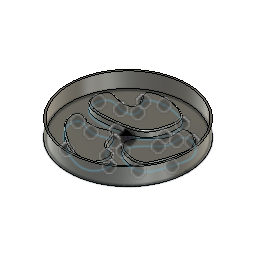
TreeCircleNatural (Autodesk Fusion 360 design; units mm, degrees)
part number: 2026-04-19-12-51-08-975
Autodesk Fusion 360 part; units mm, degrees
sketch "Sketch1" plane through (0, 0, 0) normal (0, 0, 1) x (1, 0, 0)
  circle A0 centre (0, 0) radius 49.5
  circle A1 centre (0, 0) radius 51
  spline S0 degree 5 poles (-8.877426, 39.65922) (-9.821768, 39.602929) (-11.679978, 39.421488) (-14.327292, 38.942346) (-17.354011, 37.914724) (-19.766072, 36.123006) (-20.47548, 33.984554) (-19.509504, 31.627397) (-17.465934, 29.079171) (-15.289166, 26.333804) (-13.947888, 23.4551) (-14.174667, 20.647723) (-16.111086, 18.392073) (-19.407676, 17.242742) (-23.484994, 17.496021) (-27.731291, 18.922825) (-31.751181, 20.409062) (-35.299448, 20.440773) (-38.087025, 18.002518) (-39.766856, 12.861128) (-39.522082, 7.230355) (-37.012223, 2.740009) (-32.437721, -0.082363) (-26.301826, -1.236337) (-19.307435, -1.150796) (-12.19163, -0.372936) (-5.599879, 0.626949) (0.088492, 1.75897) (4.753453, 3.267551) (8.436375, 5.503794) (11.276045, 8.784755) (13.420412, 13.149702) (14.974017, 18.315391) (15.867055, 23.150729) (16.029964, 27.116416) (15.41933, 30.175326) (14.008136, 32.541013) (11.793651, 34.522624) (8.79516, 36.29244) (5.06737, 37.83763) (0.723079, 39.047266) (-3.092365, 39.618645) (-6.01393, 39.759234) (-7.933085, 39.715511) (-8.877426, 39.65922) knots 0 0 0 0 0 0 0.025 0.05 0.075 0.1 0.125 0.15 0.175 0.2 0.225 0.25 0.275 0.3 0.325 0.35 0.375 0.4 0.425 0.45 0.475 0.5 0.525 0.55 0.575 0.6 0.625 0.65 0.675 0.7 0.725 0.75 0.775 0.8 0.825 0.85 0.875 0.9 0.925 0.95 0.975 1 1 1 1 1 1
  line L0 (-37.08953, 22.802825) -> (-41.022518, 5.322875)
  spline S1 degree 5 poles (30.28005, 24.422841) (31.299478, 24.113084) (33.404307, 23.303313) (36.563092, 21.566524) (39.896173, 18.51425) (42.110967, 13.869244) (42.401437, 8.78793) (41.377108, 3.541206) (39.758049, -1.635104) (38.151591, -6.542624) (36.684186, -10.981549) (35.143395, -14.764183) (33.154866, -17.725832) (30.355367, -19.738024) (26.547752, -20.719845) (21.913278, -20.65384) (16.980308, -19.58594) (12.433425, -17.615074) (8.969748, -14.886634) (7.140601, -11.584516) (7.187933, -7.925235) (8.911605, -4.148619) (11.824631, -0.477836) (15.276677, 2.915714) (18.591556, 5.953834) (21.189955, 8.681413) (22.739104, 11.327081) (23.195513, 14.187139) (22.85993, 17.411819) (22.344882, 20.879388) (22.780553, 23.898844) (24.722709, 25.186349) (27.287739, 25.161859) (29.260622, 24.732599) (30.28005, 24.422841) knots 0 0 0 0 0 0 0.03333333 0.06666667 0.1 0.13333333 0.16666667 0.2 0.23333333 0.26666667 0.3 0.33333333 0.36666667 0.4 0.43333333 0.46666667 0.5 0.53333333 0.56666667 0.6 0.63333333 0.66666667 0.7 0.73333333 0.76666667 0.8 0.83333333 0.86666667 0.9 0.93333333 0.96666667 1 1 1 1 1 1
  spline S2 degree 5 poles (-33.576909, -9.290298) (-33.969748, -9.659312) (-34.659811, -10.558512) (-35.36299, -12.343339) (-35.440825, -15.283213) (-33.886736, -19.604481) (-30.604097, -24.278353) (-25.705336, -29.101772) (-19.469232, -33.801749) (-12.34481, -37.998719) (-4.958901, -41.080908) (1.962757, -42.355162) (7.715664, -41.336105) (11.713045, -37.89716) (13.614982, -32.692861) (13.394601, -26.978862) (11.562426, -23.952084) (8.754108, -23.41617) (5.620535, -23.444427) (2.770664, -21.964101) (0.722426, -18.798682) (-0.66184, -14.715706) (-1.83761, -10.862708) (-3.375564, -8.357041) (-5.716624, -7.819666) (-8.925643, -8.884582) (-12.793493, -10.583509) (-16.972971, -11.818442) (-21.093815, -11.769052) (-24.902504, -10.401741) (-28.33532, -8.694301) (-30.739081, -8.010128) (-32.302781, -8.344424) (-33.184071, -8.921283) (-33.576909, -9.290298) knots 0 0 0 0 0 0 0.03333333 0.06666667 0.1 0.13333333 0.16666667 0.2 0.23333333 0.26666667 0.3 0.33333333 0.36666667 0.4 0.43333333 0.46666667 0.5 0.53333333 0.56666667 0.6 0.63333333 0.66666667 0.7 0.73333333 0.76666667 0.8 0.83333333 0.86666667 0.9 0.93333333 0.96666667 1 1 1 1 1 1
  line L1 (-31.025315, -6.893445) -> (-36.128504, -11.687151)
  line L2 (11.15425, 5.543411) -> (17.541544, 27.499735)
  line L3 (24.004603, 26.329664) -> (36.555498, 22.516019)
  line L4 (13.802717, -36.853231) -> (12.674383, -21.722999)
  line L5 (11.442123, -26.493674) -> (-2.929289, -18.509556)
  point P0 (-20.020894, 33.541238)
  point P1 (-14.249171, 22.71943)
  point P2 (-24.229318, 17.928959)
  point P3 (-39.056024, 14.06285)
  point P4 (-10, 0)
  point P5 (14.347897, 16.521573)
  point P6 (12.894833, 33.408567)
  point P7 (39.565265, -2.174221)
  point P8 (28.703333, -19.997899)
  point P9 (7.727394, -11.913422)
  point P10 (19.198494, 6.672351)
  point P11 (22.676376, 18.844937)
  point P12 (-17.407956, -34.854724)
  point P13 (13.23855, -29.288115)
  point P14 (4.256417, -22.501615)
  point P15 (-3.727701, -8.729012)
  point P16 (-19.927675, -11.586528)
  dimension "d25" = 99
  dimension "d26" = 1.5
  constraint coincident A0.centre A1.centre
  measures "d25" diameter of A0
extrude "Extrude1" add sketch "Sketch1" along normal blind 1.5 contours A0 picked at (22.700219, -29.932973)
extrude "Extrude2" add sketch "Sketch1" along normal blind 14.5 contours A1 picked at (13.665249, 48.484939)
extrude "Extrude3" add sketch "Sketch1" along normal blind 6.5 contours S0 | S1 | S2 picked at (1.944708, 27.635372) picked at (24.026795, -11.08375) picked at (-9.959647, -21.336037)
fillet "Fillet1" radius 1 3 faces at (1.944708, 27.635372, 6.5) (-9.959647, -21.336037, 6.5) (24.026795, -11.08375, 6.5)
sketch "Sketch2" plane through (0, 0, 6.5) normal (0, 0, 1) x (-1, 0, 0)
  spline S0 degree 3 poles (32.892249, 10.01916) (32.639104, 9.781367) (32.341545, 9.589308) (31.691299, 9.345674) (31.342184, 9.294593) (30.743797, 9.296004) (30.49299, 9.322423) (29.625931, 9.471285) (29.026495, 9.672167) (27.849945, 10.117946) (27.272335, 10.366643) (25.294265, 11.212513) (23.878664, 11.80168) (21.546997, 12.392487) (20.677982, 12.538232) (18.46681, 12.692028) (17.120881, 12.584062) (14.890425, 12.144926) (13.987278, 11.893609) (12.248694, 11.323428) (11.41373, 11.008363) (9.929536, 10.43333) (9.278408, 10.175064) (8.148979, 9.76338) (7.674925, 9.600846) (6.778569, 9.352594) (6.357253, 9.257588) (5.532375, 9.18223) (5.124765, 9.195114) (4.41354, 9.441239) (4.118294, 9.656287) (3.536589, 10.275427) (3.281545, 10.705885) (2.804958, 11.645419) (2.593993, 12.165124) (2.200354, 13.211421) (2.018875, 13.739079) (1.453517, 15.398765) (1.074518, 16.537048) (0.261691, 18.528471) (-0.144707, 19.395236) (-1.107036, 20.975227) (-1.655001, 21.694555) (-2.696808, 22.668435) (-3.121104, 22.99178) (-4.130063, 23.594496) (-4.72877, 23.846987) (-5.979413, 24.207212) (-6.628967, 24.311458) (-7.680977, 24.441657) (-8.086073, 24.483043) (-8.93008, 24.602249) (-9.370487, 24.682123) (-10.108902, 24.949236) (-10.414242, 25.111722) (-10.986027, 25.581338) (-11.234128, 25.902828) (-11.513583, 26.39926) (-11.588244, 26.552941) (-11.849781, 27.16373) (-11.98276, 27.642119) (-12.21242, 28.812619) (-12.270911, 29.512694) (-12.282759, 31.574676) (-12.085237, 32.942382) (-11.445065, 34.912408) (-11.16414, 35.565374) (-10.224436, 37.222913) (-9.43084, 38.15383) (-8.05765, 39.18667) (-7.612556, 39.460254) (-6.600386, 39.965441) (-6.025938, 40.181437) (-3.993743, 40.74869) (-2.476548, 40.843687) (0.355687, 40.683378) (1.680887, 40.464865) (4.284036, 39.850757) (5.563345, 39.454065) (9.108573, 38.16322) (11.322048, 37.131678) (15.686284, 34.78594) (17.835004, 33.459421) (21.614899, 30.828326) (23.268987, 29.560669) (26.132044, 27.097827) (27.369002, 25.930652) (29.480277, 23.660861) (30.380389, 22.583295) (31.817453, 20.550308) (32.390717, 19.620621) (33.268333, 17.844079) (33.602897, 17.011668) (34.023726, 15.484375) (34.148777, 14.800728) (34.217615, 13.580035) (34.196221, 13.04539) (34.042798, 12.14074) (33.942707, 11.765819) (33.673361, 11.088558) (33.512988, 10.782514) (33.188628, 10.32938) (33.048471, 10.165908) (32.892249, 10.01916) knots -1 -1 -1 -1 -0.99182189 -0.99182189 -0.98364947 -0.98364947 -0.97773188 -0.97773188 -0.96292991 -0.96292991 -0.94812793 -0.94812793 -0.9122018 -0.9122018 -0.89153292 -0.89153292 -0.86000425 -0.86000425 -0.83799615 -0.83799615 -0.81692118 -0.81692118 -0.80042749 -0.80042749 -0.78867008 -0.78867008 -0.77852683 -0.77852683 -0.7691627 -0.7691627 -0.76080474 -0.76080474 -0.74915897 -0.74915897 -0.73599842 -0.73599842 -0.72283787 -0.72283787 -0.694649 -0.694649 -0.67215453 -0.67215453 -0.65106978 -0.65106978 -0.63857965 -0.63857965 -0.6233961 -0.6233961 -0.60795231 -0.60795231 -0.598338 -0.598338 -0.58787811 -0.58787811 -0.57985207 -0.57985207 -0.57045558 -0.57045558 -0.56643794 -0.56643794 -0.55480857 -0.55480857 -0.53835115 -0.53835115 -0.50623272 -0.50623272 -0.48957313 -0.48957313 -0.46136545 -0.46136545 -0.449114 -0.449114 -0.43473219 -0.43473219 -0.39943352 -0.39943352 -0.36793594 -0.36793594 -0.33643836 -0.33643836 -0.27909649 -0.27909649 -0.21970043 -0.21970043 -0.17067231 -0.17067231 -0.1306277 -0.1306277 -0.09768056 -0.09768056 -0.07202608 -0.07202608 -0.05100159 -0.05100159 -0.03472756 -0.03472756 -0.02220907 -0.02220907 -0.01312194 -0.01312194 -0.0050469 -0.0050469 0 0 0 0
  circle A0 centre (4.124558, 14.101561) radius 35
  dimension "d35" = 70
  measures "d35" diameter of A0
extrude "Extrude4" cut sketch "Sketch2" along normal blind 1
pattern_linear "R-Pattern1" count 5 spacing 2 along (0, 0, 1) of "Extrude4"
equation "WallThickness = 1.5 mm"
equation "ChamberHeight = 5 mm"
equation "InternalConnectionTubeThickness = 3 mm"
equation "InternalTubeFillet = 1 mm"
equation "ChamberFillet = 1 mm"
equation "TopSkinMaxThickness = 8 mm"
equation "BaseSkinMaxThickness = 8 mm"
equation "PipeHoleDiameter = 1.5 mm"
equation "TotalTopSkinHeigth = WallThickness + ChamberHeight + TopSkinMaxThickness"
equation "TotalBaseSkinHeigth = WallThickness + BaseSkinMaxThickness"
equation "Tolerances = 0.2 mm"
equation "OrganCoverExtraMargin = 10 mm"
equation "OrganCoverAdaperThickness = 2 mm"
equation "NumberOfToleranceDifferencesOrganCoverToHole = 4"
equation "OrganThicknessBelowCover = 4 mm"
equation "OrganFillet = 1 mm"
equation "CircleDiameter = 99 mm"
equation "d25 = CircleDiameter"
equation "d26 = WallThickness"
equation "d27 = WallThickness"
equation "d29 = TotalTopSkinHeigth"
equation "d31 = ChamberHeight + WallThickness"
equation "d34 = ChamberFillet"
